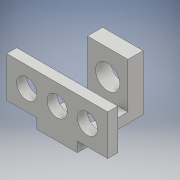
# Autodesk Inventor part: P3-9
Saved by Autodesk Inventor 2017 (Build 210142000, 142)
## iProperties
Created: 2017-02-12
Part Number: P3-9
Material: Generic
Document SubType Name: Modeling
Designer: Schaffel
Density: 1 g/cm^3
Appearance: Default
Author: Schaffel
Autodesk Inventor part; units mm, degrees
ref_plane "YZ Plane" through (0, 0, 0) normal (1, 0, 0) x (0, 1, 0)
ref_plane "XZ Plane" through (0, 0, 0) normal (0, 1, 0) x (-1, 0, 0)
ref_plane "XY Plane" through (0, 0, 0) normal (0, 0, 1) x (1, 0, 0)
sketch "Sketch1" plane through (0, 0, 0) normal (0, 0, 1) x (1, 0, 0)
  line L0 (0, 0) -> (100, 0)
  line L1 (100, 0) -> (100, 10)
  line L2 (70, 65) -> (30, 65)
  line L3 (0, 10) -> (0, 0)
  line L4 (0, 10) -> (100, 10)
  line L5 (30, 65) -> (30, 0)
  line L6 (70, 65) -> (70, 0)
  dimension "d0" = 100
  dimension "d1" = 10
  constraints: 14 end point, 4 perpendicular, 2 point on line, 1 horizontal
  measures "d0" distance of L0.start L0.end
  measures "d1" distance of L0.end L1.end
extrude "Extrusion1" add sketch "Sketch1" along normal blind 10 contours L5 L4 L6 L0 | L5 L2 L6 L4
sketch "Sketch2" plane through (0, 0, 10) normal (0, 0, 1) x (1, 0, 0)
  line L0 (0, 0) -> (100, 0)
  line L1 (100, 0) -> (100, 10)
  line L2 (100, 10) -> (0, 10)
  line L3 (0, 10) -> (0, 0)
  constraints: 8 end point, 3 perpendicular, 1 horizontal
extrude "Extrusion2" add sketch "Sketch2" along normal blind 40
sketch "Sketch3" plane through (0, 0, 10) normal (0, 0, 1) x (1, 0, 0)
  line L0 (70, 65) -> (30, 65) projected
  line L1 (30, 65) -> (70, 65)
  line L2 (70, 65) -> (70, 50)
  line L3 (70, 0) -> (70, 65) projected
  line L4 (70, 50) -> (30, 50)
  line L5 (30, 65) -> (30, 0) projected
  line L6 (30, 50) -> (30, 65)
  point P0 (0, 0)
  constraints: 8 end point, 2 collinear, 1 horizontal, 1 point on line
extrude "Extrusion3" add sketch "Sketch3" along normal blind 45
sketch "Sketch4" plane through (30, 65, 0) normal (0, 1, 0) x (1, 0, 0)
  circle A0 centre (20, -30) radius 12
  point P0 (-30, 0)
  constraints: 1 centre point
extrude "Extrusion4" cut sketch "Sketch4" against normal blind 15
sketch "Sketch5" plane through (0, 0, 10) normal (0, 0, 1) x (1, 0, 0)
  circle A0 centre (50, 30) radius 12
  point P0 (0, 0)
  constraints: 1 centre point
extrude "Extrusion5" cut sketch "Sketch5" against normal blind 10
sketch "Sketch6" plane through (30, 0, 0) normal (0, -1, 0) x (1, 0, 0)
  circle A0 centre (-10, 30) radius 10
  circle A1 centre (20, 30) radius 10
  circle A2 centre (50, 30) radius 10
  line L0 (40, 10) -> (40, 55) projected
  point P0 (-30, 0)
  constraints: 3 centre point, 1 tangent
extrude "Extrusion6" cut sketch "Sketch6" against normal blind 10
body "Solid1"
